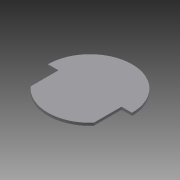
# Autodesk Inventor part: base
Saved by Autodesk Inventor 2015 (Build 190159000, 159)
## iProperties
Created: 2014-10-23
Part Number: base
Material: Generic
Document SubType Name: Modeling
Designer: Colin
Density: 1 g/cm^3
Appearance: Default
Author: Colin
Autodesk Inventor part; units mm, degrees
ref_plane "YZ Plane" through (0, 0, 0) normal (1, 0, 0) x (0, 1, 0)
ref_plane "XZ Plane" through (0, 0, 0) normal (0, 1, 0) x (-1, 0, 0)
ref_plane "XY Plane" through (0, 0, 0) normal (0, 0, 1) x (1, 0, 0)
sketch "Sketch6" plane through (0, 0, 0) normal (0, 1, 0) x (-1, 0, 0)
  circle A0 centre (0, 0) radius 50.8
  line L0 (50.8, 0) -> (38.1, 0)
  line L1 (38.1, 0) -> (38.1, 33.601)
  line L2 (-50.8, 0) -> (-38.1, 0)
  line L3 (-38.1, 0) -> (-38.1, 33.601)
  dimension "d9" = 101.6
  dimension "d10" = 12.7
  dimension "d11" = 12.7
  constraints: 8 end point, 4 point on circle, 2 horizontal, 2 perpendicular, 1 centre point, 1 coincident
  measures "d9" diameter of A0
  measures "d10" distance of L0.start L0.end
  measures "d11" distance of L2.start L2.end
extrude "Extrusion3" add sketch "Sketch6" along normal blind 3.175 contours A0 L2 L3 L1 L0
body "Solid3"
